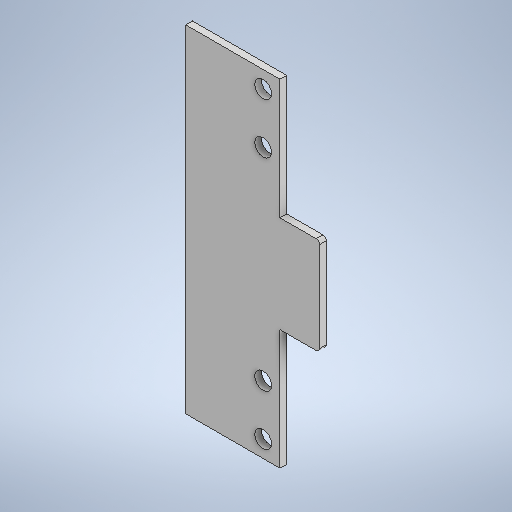
# Autodesk Inventor part: Сrane plate 2
Saved by Autodesk Inventor 2025 (Build 290162010, 162A)
## iProperties
Created: 2024-06-15
Part Number: Сrane plate 2
Material: Generic
Document SubType Name: Sheet Metal
Designer: admin
Density: 1 g/cm^3
Sheet Metal Rule: Default
Appearance: Default
Flat Pattern Width: 15.9 cm
Flat Pattern Length: 40 cm
Flat Pattern Area: 636 cm^2
Sheet Metal Width: 159,000 mm
Sheet Metal Length: 400,000 mm
Sheet Metal Area: 63600,000 mm^2
Stock Number: Кран пластина 2
Author: admin
Autodesk Inventor part; units mm, degrees
ref_plane "YZ Plane" through (0, 0, 0) normal (1, 0, 0) x (0, 1, 0)
ref_plane "XZ Plane" through (0, 0, 0) normal (0, 1, 0) x (-1, 0, 0)
ref_plane "XY Plane" through (0, 0, 0) normal (0, 0, 1) x (1, 0, 0)
sketch "Sketch1" plane through (0, 0, 0) normal (0, 1, 0) x (-1, 0, 0)
  line L0 (56, -200) -> (-56, -200)
  line L1 (-56, -200) -> (-56, 200)
  line L2 (-56, 200) -> (56, 200)
  line L3 (56, 200) -> (56, -200)
  line L4 (56, -200) -> (-56, 200) construction
  line L5 (-56, -200) -> (56, 200) construction
  line L6 (-56, 57.5) -> (-103, 57.5)
  line L7 (-103, 57.5) -> (-103, -57.5)
  line L8 (-103, -57.5) -> (-56, -57.5)
  point P0 (0, 0)
  point P1 (0, 0)
  point P2 (-103, 0)
  point P3 (-56, 0)
  dimension "d16" = 112
  dimension "d17" = 400
  dimension "d24" = 47
  dimension "d25" = 115
  measures "d16" distance of L1.end L2.end
  measures "d17" distance of L0.end L1.end
  measures "d24" distance between parallel lines of L1 L7
  measures "d25" distance of L6.end L7.end
extrude "Plate1" add sketch "Sketch1" along normal blind 8
sketch "Sketch2" plane through (0, 0, 0) normal (0, -1, 0) x (1, 0, 0)
  line L0 (36, 180) -> (36, -180) construction
  line L1 (-56, -200) -> (56, -200) projected
  line L2 (56, -200) -> (56, -57.5) projected
  line L3 (56, 200) -> (-56, 200) projected
  line L4 (-56, 200) -> (-56, -200) projected
  line L5 (103, -57.5) -> (56, -57.5) projected
  line L6 (103, 57.5) -> (103, -57.5) projected
  line L7 (56, 57.5) -> (103, 57.5) projected
  line L8 (56, 57.5) -> (56, 200) projected
  point P0 (36, 0)
  point P1 (36, 0)
  point P2 (0, 0)
  point P3 (36, 120)
  point P4 (36, -120)
  dimension "d19" = 20
  dimension "d20" = 20
  dimension "d21" = 360
  dimension "d22" = 120
  dimension "d23" = 120
  constraints: 2 coincident, 2 end point, 2 point on line, 1 horizontal alignment, 1 midpoint, 1 vertical
  measures "d19" distance between parallel lines of L2 L0
  measures "d20" distance from line of L0.start L3
  measures "d21" distance of L0.start L0.end
  measures "d22" distance of point (36, 0) point (36, -120)
  measures "d23" distance of point (36, 0) point (36, 120)
hole "Hole1" at (36, 0, 180) at (36, 0, -180) at (36, 0, -120) at (36, 0, 120) direction (0, 1, 0) diameter 20 end through all
fillet "Fillet1" radius 4 2 edges at (103, 4, 57.5) (103, 4, -57.5)
equation "\"d20\" = d19"
equation "\"d22\" = d23"
equation "\"d3\" = d19"
equation "\"d8\" = Thickness"
equation "\"d2\" = Thickness"
equation "\"BendRadius\" = Thickness"
equation "\"BendReliefWidth\" = Thickness"
equation "\"BendReliefDepth\" = 0.5 * Thickness"
equation "\"CornerReliefSize\" = 4 * Thickness"
equation "\"MinimumRemnant\" = 2 * Thickness"
equation "\"TransitionRadius\" = BendRadius"
equation "\"JacobiRadiusSize\" = BendRadius"
equation "\"GapSize\" = Thickness"
equation "\"Thickness\" = 8"
body "Solid1"
